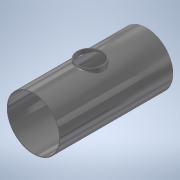
# Autodesk Inventor part: Trójnik red. krótki  Ø85 41 85 s=1,5 L=180
Saved by Autodesk Inventor 2020 (Build 240168000, 168)
## iProperties
RuleStatus: InUse
Created: 2022-03-21
Part Number: Trójnik red. krótki  Ø85 41 85 s=1,5 L=180
Material: 304
Description: Trójnik red. krótki  Ø85 41 85 s=1,5 L=180
Document SubType Name: Modelowanie
Designer: Radosław
Density: 8 g/cm^3
Sheet Metal Rule: 1,5
Sheet Metal Width: 0,000 mm
Sheet Metal Length: 0,000 mm
Sheet Metal Area: 0,000 mm^2
Appearance: Częściowo polerowany(1)
Author: Radosław
Autodesk Inventor part; units mm, degrees
ref_plane "YZ Plane" through (0, 0, 0) normal (1, 0, 0) x (0, 1, 0)
ref_plane "XZ Plane" through (0, 0, 0) normal (0, 1, 0) x (-1, 0, 0)
ref_plane "XY Plane" through (0, 0, 0) normal (0, 0, 1) x (1, 0, 0)
sketch "Szkic8" plane through (0, 0, 0) normal (0, 1, 0) x (-1, 0, 0)
  circle A0 centre (0, 0) radius 42.5
  circle A1 centre (0, 0) radius 41
  dimension "d53" = 85
  dimension "d54" = 1.5
  constraints: 2 centre point, 2 coincident
  measures "d53" diameter of A0
  measures "d54" radial gap between concentric circles of A0 A1
extrude "Wyciągnięcie proste2" add sketch "Szkic8" along normal mid plane 180
sketch "Szkic13" plane through (0, 0, 0) normal (0, 0, 1) x (1, 0, 0)
  circle A0 centre (0, 0) radius 20.5
  circle A1 centre (0, 0) radius 19
  dimension "d67" = 41
  dimension "d68" = 1.5
  constraints: 2 centre point, 1 coincident
  measures "d67" diameter of A0
  measures "d68" radial gap between concentric circles of A0 A1
extrude "Wyciągnięcie proste6" add sketch "Szkic13" along normal blind 45
sketch "Szkic14" plane through (0, 0, 45) normal (0, 0, 1) x (1, 0, 0)
  circle A0 centre (0, 0) radius 19 projected
extrude "Wyciągnięcie proste7" cut sketch "Szkic14" against normal blind 45
sketch "Szkic15" plane through (0, -90, 0) normal (0, -1, 0) x (1, 0, 0)
  circle A0 centre (0, 0) radius 41 projected
extrude "Wyciągnięcie proste8" cut sketch "Szkic15" against normal blind 180
fillet "Zaokrąglenie3" radius 1.5 2 edges at (0.0244, 20.5, 42.5) (-0.0252, -20.5, 42.5)
fillet "Zaokrąglenie4" radius 3 2 edges at (-0.0038, -19, 41) (0.0034, 19, 41)
equation "\"d53\" = OD"
equation "\"d54\" = THK"
equation "\"d55\" = L1"
equation "\"d67\" = OD2"
equation "\"d68\" = THK"
equation "\"d69\" = L2"
equation "\"d71\" = L2"
equation "\"d73\" = L1"
equation "\"d75\" = THK"
equation "\"d76\" = 2 * THK"
equation "\"SzerokośćGięciaPodcięcia\" = Grubość"
equation "\"RozmiarPodcięciaNarożnika\" = 4 * Grubość"
equation "\"PromieńPrzejścia\" = PromieńGięcia"
equation "\"Rozmiar_promienia_Jacobiego\" = PromieńGięcia"
equation "\"Wielk_odstępu\" = Grubość"
equation "\"d2\" = PromieńGięcia"
equation "\"d23\" = PromieńGięcia"
equation "\"OD\" = 85"
equation "\"THK\" = 1.5"
equation "\"L1\" = 180"
equation "\"L2\" = 45"
equation "\"OD2\" = 41"
equation "\"Grubość\" = 1.5"
equation "\"PromieńGięcia\" = 3"
